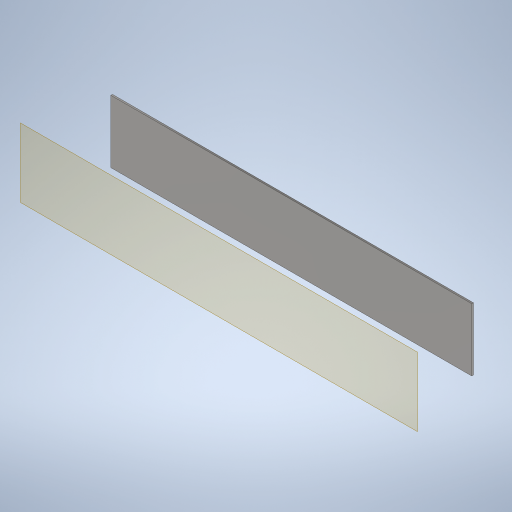
# Autodesk Inventor part: Fechamento
Saved by Autodesk Inventor 2024.2 (Build 282272000, 272)
## iProperties
Created: 2024-05-06
Part Number: Fechamento
Material: Steel, Alloy
Document SubType Name: Modeling
Designer: 082220005
Density: 7.73 g/cm^3
Appearance: Semi-Polished
Author: 082220005
Autodesk Inventor part; units mm, degrees
ref_plane "YZ Plane" through (0, 0, 0) normal (1, 0, 0) x (0, 1, 0)
ref_plane "XZ Plane" through (0, 0, 0) normal (0, 1, 0) x (-1, 0, 0)
ref_plane "XY Plane" through (0, 0, 0) normal (0, 0, 1) x (1, 0, 0)
sketch "Sketch1" plane through (0, 0, 0) normal (0, 0, 1) x (1, 0, 0)
  line L0 (0, 0) -> (75, 0)
  line L1 (75, 0) -> (75, 13)
  line L2 (75, 13) -> (0, 13)
  line L3 (0, 13) -> (0, 0)
  dimension "d0" = 75
  dimension "d1" = 13
  constraints: 8 end point, 3 perpendicular, 1 horizontal
  measures "d0" distance of L0.start L0.end
  measures "d1" distance of L0.end L1.end
extrude "Extrusion1" add sketch "Sketch1" along normal blind 0.3556
ref_plane "Work Plane1" through (0, 0, 15.3556) normal (0, 0, 1) x (1, 0, 0)
body "Solid1"
